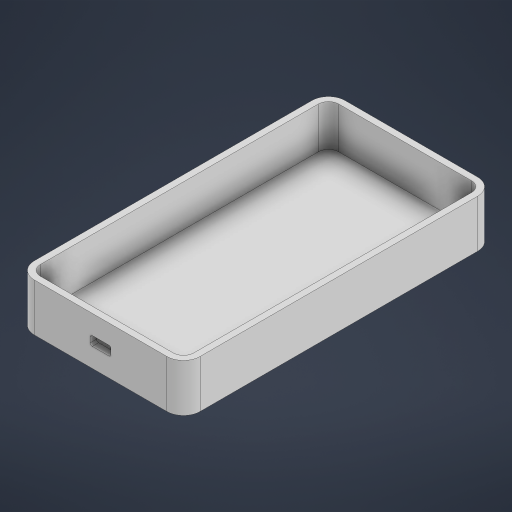
# Autodesk Inventor part: csing
Saved by Autodesk Inventor 2024 (Build 280153000, 153)
## iProperties
Created: 2025-06-11
Part Number: csing
Material: Generic
Document SubType Name: Modeling
Designer: ASUS
Density: 1 g/cm^3
Appearance: Default
Author: ASUS
Autodesk Inventor part; units mm, degrees
ref_plane "YZ Plane" through (0, 0, 0) normal (1, 0, 0) x (0, 1, 0)
ref_plane "XZ Plane" through (0, 0, 0) normal (0, 1, 0) x (-1, 0, 0)
ref_plane "XY Plane" through (0, 0, 0) normal (0, 0, 1) x (1, 0, 0)
sketch "Sketch1" plane through (0, 0, 0) normal (0, 1, 0) x (-1, 0, 0)
  line L0 (26.7027, -40.183) -> (-37.2973, -40.183)
  line L1 (-45.2973, -32.183) -> (-45.2973, 101.817)
  line L2 (-37.2973, 109.817) -> (26.7027, 109.817)
  line L3 (34.7027, 101.817) -> (34.7027, -32.183)
  arc A0 (26.7027, -40.183) -> (34.7027, -32.183) centre (26.7027, -32.183) ccw
  arc A1 (-45.2973, -32.183) -> (-37.2973, -40.183) centre (-37.2973, -32.183) ccw
  arc A2 (-37.2973, 109.817) -> (-45.2973, 101.817) centre (-37.2973, 101.817) ccw
  arc A3 (34.7027, 101.817) -> (26.7027, 109.817) centre (26.7027, 101.817) ccw
  point P0 (0, 0)
  point P1 (-45.2973, 109.817)
  point P2 (-45.2973, -40.183)
  point P3 (34.7027, 109.817)
  dimension "d0" = 80
  dimension "d1" = 150
  dimension "d2" = 8
  constraints: 8 end point, 8 point on circle, 8 tangent, 6 point on line, 4 centre point, 3 equal radius, 2 parallel, 1 horizontal, 1 perpendicular
  measures "d0" distance of point (-45.297, 109.817) point (34.703, 109.817)
  measures "d1" distance of point (-45.297, -40.183) point (-45.297, 109.817)
  measures "d2" radius of A0
extrude "Extrusion1" add sketch "Sketch1" along normal blind 3
sketch "Sketch2" plane through (0, 3, 0) normal (0, 1, 0) x (1, 0, 0)
  line L0 (-26.7027, 40.183) -> (37.2973, 40.183)
  line L1 (45.2973, 32.183) -> (45.2973, -101.817)
  line L2 (37.2973, -109.817) -> (-26.7027, -109.817)
  line L3 (-34.7027, -101.817) -> (-34.7027, 32.183)
  arc A0 (-26.7027, 40.183) -> (-34.7027, 32.183) centre (-26.7027, 32.183) ccw
  arc A1 (45.2973, 32.183) -> (37.2973, 40.183) centre (37.2973, 32.183) ccw
  arc A2 (37.2973, -109.817) -> (45.2973, -101.817) centre (37.2973, -101.817) ccw
  arc A3 (-34.7027, -101.817) -> (-26.7027, -109.817) centre (-26.7027, -101.817) ccw
  line L4 (37.2973, 37.183) -> (-26.7027, 37.183)
  arc A4 (-26.7027, 37.183) -> (-31.7027, 32.183) centre (-26.7027, 32.183) ccw
  line L5 (-31.7027, 32.183) -> (-31.7027, -101.817)
  arc A5 (-31.7027, -101.817) -> (-26.7027, -106.817) centre (-26.7027, -101.817) ccw
  line L6 (-26.7027, -106.817) -> (37.2973, -106.817)
  arc A6 (37.2973, -106.817) -> (42.2973, -101.817) centre (37.2973, -101.817) ccw
  line L7 (42.2973, -101.817) -> (42.2973, 32.183)
  arc A7 (42.2973, 32.183) -> (37.2973, 37.183) centre (37.2973, 32.183) ccw
  point P0 (0, 0)
  dimension "d5" = 8
  dimension "d6" = 3
  constraints: 16 end point, 16 point on circle, 8 centre point, 8 tangent, 4 parallel, 3 equal radius, 2 perpendicular, 1 horizontal, 7 other
  measures "d5" radius of A0
  measures "d6" distance between parallel lines of L0 L4
extrude "Extrusion2" add sketch "Sketch2" along normal blind 20
sketch "Sketch3" plane through (-26.7027, 0, 109.817) normal (0, 0, 1) x (1, 0, 0)
  line L0 (64, 0) -> (0, 0) projected
  line L1 (32, 0) -> (32, 11.5)
  line L2 (28, 13.75) -> (36, 13.75)
  line L3 (37, 12.75) -> (37, 10.25)
  line L4 (36, 9.25) -> (28, 9.25)
  line L5 (27, 10.25) -> (27, 12.75)
  line L6 (27, 13.75) -> (37, 9.25) construction
  line L7 (37, 13.75) -> (27, 9.25) construction
  arc A0 (28, 13.75) -> (27, 12.75) centre (28, 12.75) ccw
  arc A1 (37, 12.75) -> (36, 13.75) centre (36, 12.75) ccw
  arc A2 (36, 9.25) -> (37, 10.25) centre (36, 10.25) ccw
  arc A3 (27, 10.25) -> (28, 9.25) centre (28, 10.25) ccw
  point P0 (26.7027, 0)
  dimension "d9" = 11.5
  dimension "d10" = 10
  dimension "d11" = 4.5
  dimension "d14" = 1
  constraints: 14 end point, 8 point on circle, 8 point on line, 8 tangent, 4 centre point, 3 equal radius, 3 midpoint, 2 parallel, 1 horizontal, 1 perpendicular, 1 vertical
  measures "d9" distance of L1.start L1.end
  measures "d10" distance of L6.end L7.end
  measures "d11" distance of L7.start L6.end
  measures "d14" radius of A0
extrude "Extrusion3" cut sketch "Sketch3" against normal blind 3
body "Solid1"
